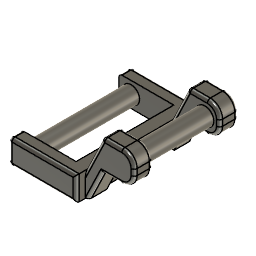
Roller Arm (Autodesk Fusion 360 design; units mm, degrees)
part number: 2026-03-22-23-28-42-444
Autodesk Fusion 360 part; units mm, degrees
sketch "Sketch3" plane through (0, -13.97, 0) normal (0, -1, 0) x (1, 0, 0)
  line L0 (0, 10.16) -> (10.16, 10.16)
  line L1 (10.16, 10.16) -> (10.16, 20.32)
  line L2 (10.16, 20.32) -> (0, 20.32)
  line L3 (5.08, 20.32) -> (12.4091, 35.56)
  line L4 (12.4091, 35.56) -> (25.4, 35.56)
  line L5 (25.4, 35.56) -> (25.4, 22.86)
  line L6 (25.4, 22.86) -> (12.4576, 22.86)
  line L7 (12.4576, 22.86) -> (6.35, 10.16)
  line L8 (5.08, 20.32) -> (0, 20.32)
  line L9 (0, 10.16) -> (6.35, 10.16)
  line L10 (0, 20.32) -> (0, 10.16)
  line L11 (-25.4, 0) -> (0, 0)
  line L12 (0, 20.32) -> (0, 10.16)
  dimension "d22" = 25.4
  dimension "d23" = 22.86
  dimension "d24" = 12.7
  constraint perpendicular L4 L5
  constraint perpendicular L5 L6
  constraint parallel L3 L7
  constraint midpoint L2 L3.start
  constraint coincident L2.end L8.end
  constraint coincident L0.start L9.start
  measures "d22" distance of L5 L10
  measures "d23" distance of L6 L11
  measures "d24" distance of L4 L6
extrude "Extrude3" add sketch "Sketch3" along normal blind 7.62 contours L0 L1 L2 L7 L8 L9 L10 L12 | L1 L2 L3 L4 L5 L6 L7 makes body 1
mirror "Mirror1" about plane through (0, 0, 0) normal (0, 1, 0) of "Extrude3" makes body 2
sketch "Sketch4" plane through (0, -13.97, 0) normal (0, 1, 0) x (-1, 0, 0)
  line L0 (0, 20.32) -> (-5.08, 20.32)
  line L1 (-5.08, 20.32) -> (-12.4091, 35.56)
  line L2 (-12.4091, 35.56) -> (-25.4, 35.56)
  line L3 (-25.4, 35.56) -> (-25.4, 22.86)
  line L4 (-25.4, 22.86) -> (-12.4576, 22.86)
  line L5 (-12.4576, 22.86) -> (-6.35, 10.16)
  circle A0 centre (-19.346, 29.21) radius 3.683
  line L6 (-32.4673, 29.21) -> (-5.1482, 29.21) construction
  line L7 (-6.35, 10.16) -> (0, 10.16)
  line L8 (0, 10.16) -> (0, 20.32)
  dimension "d19" = 7.366
  constraint perpendicular L3 L6
  constraint coincident A0.centre L6
  measures "d19" diameter of A0
extrude "Extrude4" add sketch "Sketch4" along normal up to surface (27.94 mm away) contours A0 bodies 1
sketch "Sketch9" plane through (0, -21.59, 0) normal (0, -1, 0) x (1, 0, 0)
  line L0 (6.35, 10.16) -> (12.4576, 22.86)
  line L1 (12.4576, 22.86) -> (25.4, 22.86)
  line L2 (25.4, 22.86) -> (25.4, 35.56)
  line L3 (25.4, 35.56) -> (12.4091, 35.56)
  line L4 (12.4091, 35.56) -> (5.08, 20.32)
  line L5 (5.08, 20.32) -> (0, 20.32)
  line L6 (0, 20.32) -> (0, 10.16)
  line L7 (0, 10.16) -> (6.35, 10.16)
  line L8 (0, 20.32) -> (5.08, 20.32)
  line L9 (5.08, 20.32) -> (5.08, 10.16)
  line L10 (5.08, 10.16) -> (0, 10.16)
  line L11 (0, 10.16) -> (0, 20.32)
  dimension "d57" = 5.08
  constraint horizontal L8
  constraint vertical L9
  constraint horizontal L10
  constraint vertical L11
  constraint coincident L7 L9.end
  constraint coincident L5.end L6.start
  measures "d57" distance of L9 L11
extrude "Extrude10" add sketch "Sketch9" along normal blind 3.81 contours L5 L6 L7 L8 L9 L10 L11 bodies 1
sketch "Sketch10" plane through (0, 21.59, 0) normal (0, 1, 0) x (-1, 0, 0)
  line L0 (-12.4576, 22.86) -> (-6.35, 10.16)
  line L1 (-6.35, 10.16) -> (0, 10.16)
  line L2 (0, 10.16) -> (0, 20.32)
  line L3 (0, 20.32) -> (-5.08, 20.32)
  line L4 (-5.08, 20.32) -> (-12.4091, 35.56)
  line L5 (-12.4091, 35.56) -> (-25.4, 35.56)
  line L6 (-25.4, 35.56) -> (-25.4, 22.86)
  line L7 (-25.4, 22.86) -> (-12.4576, 22.86)
  line L8 (0, 20.32) -> (-5.08, 20.32)
  line L9 (-5.08, 20.32) -> (-5.08, 10.16)
  line L10 (-5.08, 10.16) -> (0, 10.16)
  line L11 (0, 10.16) -> (0, 20.32)
  dimension "d54" = 5.08
  constraint horizontal L8
  constraint vertical L9
  constraint horizontal L10
  constraint vertical L11
  constraint coincident L1 L9.end
  constraint coincident L2.end L3.start
  measures "d54" distance of L9 L11
extrude "Extrude11" add sketch "Sketch10" along normal blind 3.81 contours L1 L2 L3 L8 L9 L10 L11 bodies 2
sketch "Sketch11" plane through (0, 0, 0) normal (-1, 0, 0) x (0, -1, 0)
  line L0 (-13.97, 10.16) -> (-13.97, 20.32)
  line L1 (-13.97, 20.32) -> (-25.4, 20.32)
  line L2 (-25.4, 20.32) -> (-25.4, 10.16)
  line L3 (-25.4, 10.16) -> (-13.97, 10.16)
  line L4 (-25.4, 20.32) -> (-20.32, 20.32)
  line L5 (-20.32, 20.32) -> (-20.32, 10.16)
  line L6 (-20.32, 10.16) -> (-25.4, 10.16)
  line L7 (-25.4, 10.16) -> (-25.4, 20.32)
  line L8 (25.4, 20.32) -> (20.32, 20.32)
  line L9 (20.32, 20.32) -> (20.32, 10.16)
  line L10 (20.32, 10.16) -> (25.4, 10.16)
  line L11 (25.4, 10.16) -> (25.4, 20.32)
  line L12 (25.4, 20.32) -> (25.4, 10.16)
  line L13 (13.97, 20.32) -> (25.4, 20.32)
  dimension "d58" = 5.08
  dimension "d59" = 10.16
  dimension "d60" = 5.08
  dimension "d61" = 10.16
  constraint horizontal L4
  constraint vertical L5
  constraint horizontal L6
  constraint vertical L7
  constraint coincident L1.end L2.start
  constraint horizontal L8
  constraint vertical L9
  constraint horizontal L10
  constraint vertical L11
  constraint collinear L11 L12
  constraint collinear L8 L13
  measures "d58" distance of L1.end L4.end
  measures "d59" distance of L1.end L2.end
  measures "d60" distance of L8.start L8.end
  measures "d61" distance of L8.start L10.end
extrude "Extrude12" add sketch "Sketch11" along normal blind 22.86 contours L1 L2 L3 L4 L5 L6 L7 | L8 L9 L10 L11 L12 L13 bodies 1 2
sketch "Sketch12" plane through (0, 20.32, 0) normal (0, -1, 0) x (1, 0, 0)
  line L0 (0, 10.16) -> (0, 20.32)
  line L1 (0, 20.32) -> (-22.86, 20.32)
  line L2 (-22.86, 20.32) -> (-22.86, 10.16)
  line L3 (-22.86, 10.16) -> (0, 10.16)
  circle A0 centre (-17.78, 15.24) radius 3.556
  dimension "d64" = 7.112
  dimension "d65" = 5.08
  dimension "d66" = 5.08
  measures "d64" diameter of A0
  measures "d65" distance of L2 A0.centre
  measures "d66" distance of L3 A0.centre
extrude "Extrude13" add sketch "Sketch12" along normal up to surface (40.64 mm away) contours A0 bodies 1 2
sketch "Sketch13" plane through (0, 13.97, 0) normal (0, -1, 0) x (1, 0, 0)
  line L0 (6.35, 10.16) -> (12.4576, 22.86)
  line L1 (12.4576, 22.86) -> (25.4, 22.86)
  line L2 (25.4, 22.86) -> (25.4, 35.56)
  line L3 (25.4, 35.56) -> (12.4091, 35.56)
  line L4 (12.4091, 35.56) -> (5.08, 20.32)
  line L5 (5.08, 20.32) -> (0, 20.32)
  line L6 (0, 20.32) -> (0, 10.16)
  line L7 (0, 10.16) -> (6.35, 10.16)
  circle A0 centre (19.346, 29.21) radius 3.683
  line L8 (5.08, 20.32) -> (0, 20.32)
  line L9 (0, 20.32) -> (0, 10.16)
  line L10 (0, 10.16) -> (5.08, 10.16)
  line L11 (5.08, 10.16) -> (5.08, 20.32)
  constraint horizontal L8
  constraint vertical L9
  constraint horizontal L10
  constraint vertical L11
  constraint coincident L6.end L7.start
  constraint coincident L4.end L5.start
extrude "Extrude14" add sketch "Sketch13" along normal up to surface (27.94 mm away) contours L5 L6 L7 L8 L9 L10 L11 bodies 1
fillet "Fillet5" radius 5.08 4 edges at (25.4, 17.78, 35.56) (25.4, 17.78, 22.86) (25.4, -17.78, 35.56) (25.4, -17.78, 22.86) on bodies 1
fillet "Fillet6" radius 1.27 6 edges at (-22.86, -22.86, 20.32) (-22.86, -25.4, 15.24) (-8.89, -25.4, 20.32) (-22.86, -22.86, 10.16) (-8.89, -25.4, 10.16) (5.08, -25.4, 15.24) on bodies 1
fillet "Fillet7" radius 1.27 1 faces at (-4.2333, 25.4, 13.5467) on bodies 1
fillet "Fillet8" radius 1.27 4 edges at (-22.86, 22.225, 20.32) (-22.488, 25.028, 19.948) (-22.488, 25.028, 10.532) (-22.86, 22.225, 10.16) on bodies 1
fillet "Fillet9" radius 1.27 24 edges at (9.4038, -21.59, 16.51) (8.7446, -21.59, 27.94) (16.3888, -21.59, 22.86) (23.9121, -21.59, 24.3479) (25.4, -21.59, 29.21) (23.9121, -21.59, 34.0721) (16.3646, -21.59, 35.56) (16.3888, -13.97, 22.86) (23.9121, -13.97, 24.3479) (25.4, -13.97, 29.21) (23.9121, -13.97, 34.0721) (16.3646, -13.97, 35.56) (16.3646, 13.97, 35.56) (23.9121, 13.97, 34.0721) (25.4, 13.97, 29.21) (23.9121, 13.97, 24.3479) (16.3888, 13.97, 22.86) (16.3888, 21.59, 22.86) (23.9121, 21.59, 24.3479) (25.4, 21.59, 29.21) (23.9121, 21.59, 34.0721) (16.3646, 21.59, 35.56) (9.4038, 21.59, 16.51) (8.7446, 21.59, 27.94) on bodies 1
fillet "Fillet10" radius 1.27 8 edges at (8.4392, 13.97, 27.305) (12.2303, 14.342, 35.188) (12.4091, 17.78, 35.56) (12.643, 21.218, 35.188) (8.4392, -13.97, 27.305) (12.2303, -14.342, 35.188) (12.4091, -17.78, 35.56) (12.643, -21.218, 35.188) on bodies 1
fillet "Fillet11" radius 0.254 7 edges at (5.715, -13.97, 10.16) (5.08, 0, 10.16) (5.715, 13.97, 10.16) (6.35, 17.145, 10.16) (5.9853, 21.1725, 10.16) (6.35, -17.145, 10.16) (5.9853, -21.1725, 10.16) on bodies 1
